fingerBox_v1 (Autodesk Fusion 360 design; units mm, degrees)
Autodesk Fusion 360 part; units mm, degrees
note: some values were not read from the file. Chosen so that the rebuilt part matches the saved one: which face or edge a step refers to.
sketch "Bottom Sketch" plane through (0, 0, 0) normal (0, 0, 1) x (1, 0, 0)
  line L0 (0, 0) -> (-70, 0)
  line L1 (-70, 0) -> (-70, 5)
  line L2 (-70, 5) -> (0, 5)
  line L3 (0, 5) -> (0, 0)
  line L4 (-70, 0) -> (-60, 0)
  line L5 (-60, 0) -> (-60, 3.175)
  line L6 (-60, 3.175) -> (-50, 3.175)
  line L7 (-50, 3.175) -> (-50, 0)
  circle A0 centre (-59.2929, 2.4679) radius 1
  circle A1 centre (-50.7071, 2.4679) radius 1
  dimension "d8" = 5
  dimension "d10" = 10
  dimension "d12" = 10
  dimension "d13" = 3.175
  dimension "d14" = 3.175
  dimension "d26" = 70
  dimension "d34" = 2
  dimension "d36" = 0.7071
  dimension "d37" = 0.7071
  dimension "d38" = 0.7071
  constraint horizontal L0
  constraint vertical L1
  constraint horizontal L2
  constraint vertical L3
  constraint coincident L0.start L3.end
  constraint horizontal L4
  constraint perpendicular L4 L5
  constraint perpendicular L5 L6
  constraint perpendicular L6 L7
  constraint equal A0 A1
  constraint horizontal A0.centre A1.centre
  measures "d8" distance of L0.start L2.end
  measures "d10" distance of L0.end L4.end
  measures "d12" distance of L5.end L6.end
  measures "d13" distance of L4.end L5.end
  measures "d14" distance of L6.end L7.end
  measures "d26" distance of L1.end L2.end
  measures "d34" diameter of A0
  measures "d36" distance of L5 A0.centre
  measures "d37" distance of L6 A0.centre
  measures "d38" horizontal distance of L7.end A1.centre
extrude "Extrude1" add sketch "Bottom Sketch" along normal blind 3.175 contours L0 L1 L2 L3 L4 L5 L6 L7 A0 A1 makes body 1
pattern_linear "R-Pattern2" count 3 spacing 20 along (1, 0, 0) of 8 faces at (-58.8992, 3.3872, 2.1167) (-60.0328, 1.7952, 2.1167) (-60, 1.1739, 2.1167) (-56.1953, 3.175, 1.0583) (-50, 1.1739, 1.0583) (-49.7081, 2.4243, 2.1167) (-49.8637, 3.0052, 2.1167) (-51.3798, 3.2078, 2.1167) on bodies 1
mirror "Mirror1" about plane through (-70, 5, 0) normal (0, 1, 0) of bodies 1 makes body 2
move_body "Move1" bodies 2 to x (1, 0, 0) y (0, 1, 0) z (0, 0, 1) at (0, 2, 0)
equation "fingerWidth = 10 mm"
equation "lengthFingers = 3"
equation "length = lengthFingers * 2 * fingerWidth + fingerWidth"
equation "thickness = 3.175 mm"
equation "heightFingers = 1"
equation "height = heightFingers * 2 * fingerWidth + fingerWidth"
equation "d8 = testHeight"
equation "d10 = fingerWidth"
equation "d12 = fingerWidth"
equation "d13 = thickness"
equation "d14 = thickness"
equation "d15 = thickness"
equation "d21 = lengthFingers"
equation "d23 = -2 * fingerWidth"
equation "d26 = length"
equation "testHeight = 5 mm"
equation "d31 = toolDiameter"
equation "toolDiameter = 2 mm"
equation "d34 = toolDiameter"
equation "d36 = cornerToCenterForBone"
equation "d37 = cornerToCenterForBone"
equation "d38 = cornerToCenterForBone"
equation "cornerToCenterForBone = toolDiameter / 2 / sqrt(2)"
named bodies: "Bottom", "Bottom mirrored"
